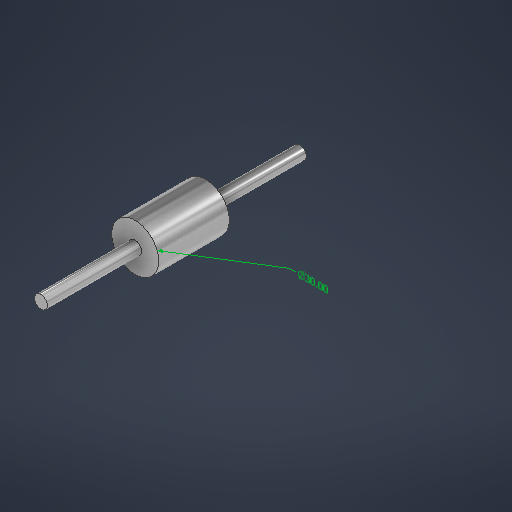
# Autodesk Inventor part: Roller with shaft
Saved by Autodesk Inventor 2026.2 (Build 302298010, 298A)
## iProperties
Created: 2026-04-16
Part Number: Roller with shaft
Material: Generic
Document SubType Name: Modeling
Designer: yassi
Density: 1 g/cm^3
Appearance: Honed
Author: yassi
## iProperties of the stored document Roller_3DPrint.ipt
Created: 2026-04-17
Part Number: Roller_3DPrint
Material: Generic
Document SubType Name: Modeling
Designer: yassi
Density: 1 g/cm^3
Appearance: Default
Author: yassi
Autodesk Inventor part; units mm, degrees
ref_plane "YZ Plane" through (0, 0, 0) normal (1, 0, 0) x (0, 1, 0)
ref_plane "XZ Plane" through (0, 0, 0) normal (0, 1, 0) x (-1, 0, 0)
ref_plane "XY Plane" through (0, 0, 0) normal (0, 0, 1) x (1, 0, 0)
sketch "Sketch1" plane through (0, 0, 0) normal (0, 0, 1) x (1, 0, 0)
  circle A0 centre (0, 0) radius 15
  circle A1 centre (0, 0) radius 4.1
  dimension "d0" = 30
  dimension "d2" = 8.2
  constraints: 2 centre point, 2 coincident
  measures "d0" diameter of A0
  measures "d2" diameter of A1
extrude "Extrusion1" add sketch "Sketch1" along normal blind 45
sketch "Sketch2" plane through (0, 0, 0) normal (0, 0, 1) x (1, 0, 0)
  point P0 (0, 0)
sketch "Sketch3" plane through (0, 0, 0) normal (0, 0, 1) x (1, 0, 0)
  point P0 (0, 0)
sketch "Sketch4" plane through (0, 0, 45) normal (0, 0, 1) x (1, 0, 0)
  circle A0 centre (0, 0) radius 4.1 projected
  circle A1 centre (0, 0) radius 4.1
  constraints: 1 centre point, 1 coincident
sketch "Sketch5" plane through (0, 0, 0) normal (0, 0, -1) x (-1, 0, 0)
  circle A0 centre (0, 0) radius 4.1
  constraints: 1 centre point, 1 coincident
extrude "Extrusion2" add sketch "Sketch5" along normal blind 60 and the other way blind 5
extrude "Extrusion3" add sketch "Sketch4" along normal blind 60
body "Solid1"
